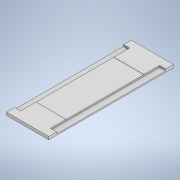
# Autodesk Inventor part: NizFlanecX_ax
Saved by Autodesk Inventor 2020.1 (Build 241239000, 239)
## iProperties
Created: 2023-01-07
Part Number: NizFlanecX_ax
Material: Типовые
Document SubType Name: Modeling
Designer: KirikDK
Density: 1 g/cm^3
Appearance: По умолчанию
Mass: 4478.88 g
Surface Area: 5356.88 cm^2
Volume: 4478.88 cm^3
Author: KirikDK
Autodesk Inventor part; units mm, degrees
ref_plane "YZ Plane" through (0, 0, 0) normal (1, 0, 0) x (0, 1, 0)
ref_plane "XZ Plane" through (0, 0, 0) normal (0, 1, 0) x (-1, 0, 0)
ref_plane "XY Plane" through (0, 0, 0) normal (0, 0, 1) x (1, 0, 0)
sketch "Эскиз1" plane through (0, 0, 0) normal (0, 1, 0) x (-1, 0, 0)
  line L0 (81.6842, 653.4737) -> (-198.3158, 653.4737)
  line L1 (-198.3158, 653.4737) -> (-198.3158, -122.5263)
  line L2 (-198.3158, -122.5263) -> (81.6842, -122.5263)
  line L3 (81.6842, -122.5263) -> (81.6842, 653.4737)
  point P0 (0, 0)
  dimension "d0" = 776
  dimension "d1" = 280
  constraints: 8 end point, 2 parallel, 1 horizontal, 1 perpendicular
  measures "d0" distance of L2.end L0.start
  measures "d1" distance of L1.end L2.end
extrude "Выдавливание1" add sketch "Эскиз1" along normal blind 20
sketch "Эскиз3" plane through (-81.6842, 0, 653.4737) normal (0, 0, 1) x (1, 0, 0)
  line L0 (292, 31) -> (240, 31)
  line L1 (240, 31) -> (240, 9)
  line L2 (240, 9) -> (292, 9)
  line L3 (292, 9) -> (292, 31)
  line L4 (0, 0) -> (280, 0) projected
  line L5 (280, 0) -> (280, 20) projected
  line L6 (-1, 23) -> (40, 23)
  line L7 (40, 23) -> (40, 9)
  line L8 (40, 9) -> (-1, 9)
  line L9 (-1, 9) -> (-1, 23)
  line L10 (0, 0) -> (0, 20) projected
  point P0 (81.6842, 0)
  dimension "d4" = 9
  dimension "d5" = 40
  dimension "d6" = 9
  dimension "d7" = 40
  constraints: 16 end point, 4 parallel, 2 horizontal, 2 perpendicular
  measures "d4" distance between parallel lines of L2 L4
  measures "d5" distance between parallel lines of L5 L1
  measures "d6" distance between parallel lines of L4 L8
  measures "d7" distance between parallel lines of L10 L7
extrude "Выдавливание2" cut sketch "Эскиз3" against normal blind 999
sketch "Эскиз4" plane through (-81.6842, 0, 653.4737) normal (0, 0, 1) x (1, 0, 0)
  point P0 (81.6842, 0)
sketch "Эскиз5" plane through (-81.6842, 0, 653.4737) normal (0, 0, 1) x (1, 0, 0)
  line L0 (280, 0) -> (280, 9) projected
  line L1 (280, 0) -> (0, 0)
  line L2 (0, 0) -> (0, 20)
  line L3 (0, 20) -> (280, 20)
  line L4 (280, 20) -> (280, 0)
  point P0 (81.6842, 0)
  dimension "d18" = 20
  constraints: 8 end point, 2 parallel, 1 horizontal, 1 perpendicular
  measures "d18" distance between parallel lines of L3 L1
extrude "Выдавливание3" add sketch "Эскиз5" along normal mid plane 52
sketch "Эскиз6" plane through (198.3158, 0, -122.5263) normal (0, 0, -1) x (-1, 0, 0)
  line L0 (0, 0) -> (280, 0) projected
  line L1 (0, 20) -> (0, 9) projected
  line L2 (280, 0) -> (0, 0)
  line L3 (0, 0) -> (0, 20)
  line L4 (0, 20) -> (280, 20)
  line L5 (280, 20) -> (280, 0)
  point P0 (198.3158, 0)
  point P1 (0, 9)
  constraints: 8 end point, 2 parallel, 1 horizontal, 1 perpendicular
extrude "Выдавливание4" add sketch "Эскиз6" along normal mid plane 52
sketch "Эскиз7" plane through (0, 20, 0) normal (0, 1, 0) x (1, 0, 0)
  line L0 (-81.6842, -627.4737) -> (198.3158, -627.4737) projected
  line L1 (198.3158, 96.5263) -> (-81.6842, 96.5263) projected
  line L2 (198.3158, 96.5263) -> (198.3158, -627.4737) projected
  line L3 (-149.6842, -265.4737) -> (289, -265.4737)
  line L4 (289, -265.4737) -> (289, -7.4737)
  line L5 (289, -7.4737) -> (-149.6842, -7.4737)
  line L6 (-149.6842, -7.4737) -> (-149.6842, -265.4737)
  line L7 (-149.6842, -265.4737) -> (289, -265.4737)
  line L8 (289, -265.4737) -> (289, -523.4737)
  line L9 (289, -523.4737) -> (-149.6842, -523.4737)
  line L10 (-149.6842, -523.4737) -> (-149.6842, -265.4737)
  point P0 (0, 0)
  dimension "d14" = 258
  dimension "d15" = 258
  constraints: 16 end point, 4 parallel, 2 horizontal, 2 perpendicular, 1 point on line
  measures "d14" distance between parallel lines of L3 L5
  measures "d15" distance between parallel lines of L9 L3
extrude "Выдавливание5" cut sketch "Эскиз7" against normal blind 1
